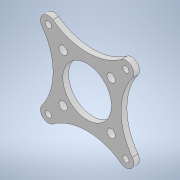
# Autodesk Inventor part: 関節3_775側_モータマウント
Saved by Autodesk Inventor 2021 (Build 250183000, 183)
## iProperties
Created: 2022-01-31
Part Number: 関節3_775側_モータマウント
Material: 一般
Document SubType Name: Modeling
Designer: hirohumi
Density: 1 g/cm^3
Appearance: 既定
Author: hirohumi
Autodesk Inventor part; units mm, degrees
ref_plane "YZ Plane" through (0, 0, 0) normal (1, 0, 0) x (0, 1, 0)
ref_plane "XZ Plane" through (0, 0, 0) normal (0, 1, 0) x (-1, 0, 0)
ref_plane "XY Plane" through (0, 0, 0) normal (0, 0, 1) x (1, 0, 0)
sketch "スケッチ1" plane through (0, 0, 0) normal (0, 0, 1) x (1, 0, 0)
  circle A0 centre (-12.3744, 12.3744) radius 2.15
  circle A1 centre (-12.3744, -12.3744) radius 2.15
  circle A2 centre (12.3744, 12.3744) radius 2.15
  circle A3 centre (12.3744, -12.3744) radius 2.15
  line L0 (12.3744, 12.3744) -> (-12.3744, 12.3744) construction
  line L1 (-12.3744, 12.3744) -> (-12.3744, -12.3744) construction
  line L2 (-12.3744, -12.3744) -> (12.3744, -12.3744) construction
  line L3 (12.3744, -12.3744) -> (12.3744, 12.3744) construction
  line L4 (12.3744, 12.3744) -> (-12.3744, -12.3744) construction
  line L5 (-12.3744, 12.3744) -> (12.3744, -12.3744) construction
  circle A4 centre (0, 0) radius 12.55
  line L6 (20, 20) -> (-20, 20) construction
  line L7 (-20, 20) -> (-20, -20) construction
  line L8 (-20, -20) -> (20, -20) construction
  line L9 (20, -20) -> (20, 20) construction
  line L10 (20, 20) -> (-20, -20) construction
  line L11 (-20, 20) -> (20, -20) construction
  circle A5 centre (-20, 20) radius 1.6
  circle A6 centre (20, 20) radius 1.6
  circle A7 centre (20, -20) radius 1.6
  circle A8 centre (-20, -20) radius 1.6
  arc A9 (-17.6484, 23.2357) -> (-23.2357, 17.6484) centre (-20, 20) ccw
  arc A10 (23.2357, 17.6484) -> (17.6484, 23.2357) centre (20, 20) ccw
  arc A11 (17.6484, -23.2357) -> (23.2357, -17.6484) centre (20, -20) ccw
  arc A12 (-23.2357, -17.6484) -> (-17.6484, -23.2357) centre (-20, -20) ccw
  circle A13 centre (0, 0) radius 17.5 construction
  arc A14 (-17.6484, 23.2357) -> (17.6484, 23.2357) centre (0, 47.5192) ccw
  arc A15 (23.2357, 17.6484) -> (23.2357, -17.6484) centre (47.5192, 0) ccw
  arc A16 (17.6484, -23.2357) -> (-17.6484, -23.2357) centre (0, -47.5192) ccw
  arc A17 (-23.2357, -17.6484) -> (-23.2357, 17.6484) centre (-47.5192, 0) ccw
  dimension "d0" = 4.3
  dimension "d1" = 4.3
  dimension "d2" = 4.3
  dimension "d3" = 4.3
  dimension "d4" = 17.5
  dimension "d5" = 25.1
  dimension "d6" = 40
  dimension "d7" = 40
  dimension "d8" = 3.2
  dimension "d9" = 3.2
  dimension "d10" = 3.2
  dimension "d11" = 3.2
  dimension "d12" = 4
  dimension "d13" = 4
  dimension "d14" = 4
  dimension "d16" = 4
  dimension "d17" = 35
  constraints: 24 end point, 18 centre point, 16 point on circle, 14 coincident, 12 tangent, 4 midpoint, 4 parallel, 3 perpendicular, 2 horizontal
  measures "d0" diameter of A0
  measures "d1" diameter of A1
  measures "d2" diameter of A2
  measures "d3" diameter of A3
  measures "d4" distance of point (0, 0) A0.centre
  measures "d5" diameter of A4
  measures "d6" distance of L8.end L7.end
  measures "d7" distance of L7.end L6.end
  measures "d8" diameter of A5
  measures "d9" diameter of A6
  measures "d10" diameter of A7
  measures "d11" diameter of A8
  measures "d12" radius of A9
  measures "d13" radius of A10
  measures "d14" radius of A11
  measures "d16" radius of A12
  measures "d17" diameter of A13
extrude "押し出し1" add sketch "スケッチ1" along normal blind 3
